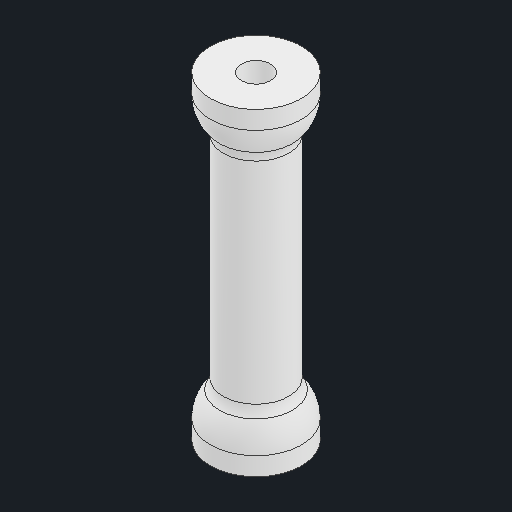
# Autodesk Inventor part: Bolt_Spacer
Saved by Autodesk Inventor 2024.3 (Build 283343010, 343A)
## iProperties
Created: 2025-03-08
Part Number: Bolt_Spacer
Material: ABS Plastic
Document SubType Name: Modeling
Designer: Owen L
Density: 1.06 g/cm^3
Appearance: Smooth - White
Mass: 6.19514 g
Surface Area: 34.7011 cm^2
Volume: 5.84448 cm^3
Author: Owen L
Autodesk Inventor part; units mm, degrees
ref_plane "YZ Plane" through (0, 0, 0) normal (1, 0, 0) x (0, 1, 0)
ref_plane "XZ Plane" through (0, 0, 0) normal (0, 1, 0) x (-1, 0, 0)
ref_plane "XY Plane" through (0, 0, 0) normal (0, 0, 1) x (1, 0, 0)
sketch "Sketch1" plane through (0, 0, 0) normal (1, 0, 0) x (0, 1, 0)
  line L0 (27.7812, 2.54) -> (0, 2.54)
  line L1 (-5.5563, 0) -> (33.3375, 0) projected
  line L2 (27.7812, 2.54) -> (27.7812, 7.9375)
  line L3 (0, 10.226) -> (0, -1.7043) projected
  line L4 (27.7812, 7.9375) -> (24.6063, 7.9375)
  line L5 (27.7812, 5.715) -> (0, 5.715)
  arc A0 (24.6063, 7.9375) -> (20.1613, 6.35) centre (24.6063, 0.9208) ccw
  arc A1 (18.3833, 5.715) -> (20.1613, 6.35) centre (18.3833, 8.5217) ccw
  point P0 (0, 0)
  dimension "d0" = 2.54
  dimension "d2" = 27.7812
  dimension "d3" = 3.175
  dimension "d5" = 3.175
  dimension "d6" = 7.62
  dimension "d9" = 7.9375
  dimension "d10" = 1.5875
  constraints: 8 end point, 4 point on circle, 4 point on line, 3 tangent, 2 centre point, 2 horizontal, 1 perpendicular, 1 vertical
  measures "d0" distance between parallel lines of L1 L0
  measures "d2" distance of L0.start L0.end
  measures "d3" distance of L2.end L4.end
  measures "d5" distance between parallel lines of L0 L5
  measures "d6" distance from line of L2 A0.end
  measures "d9" distance between parallel lines of L1 L4
  measures "d10" distance from line of A0.end L4
revolve "Revolution1" add sketch "Sketch1" angle 360 about axis through (0, 0, 0) along (0, 1, 0)
mirror "Mirror1" about plane through (0, 0, 5.715) normal (0, -1, 0) of "Revolution1"
body "Solid1"
